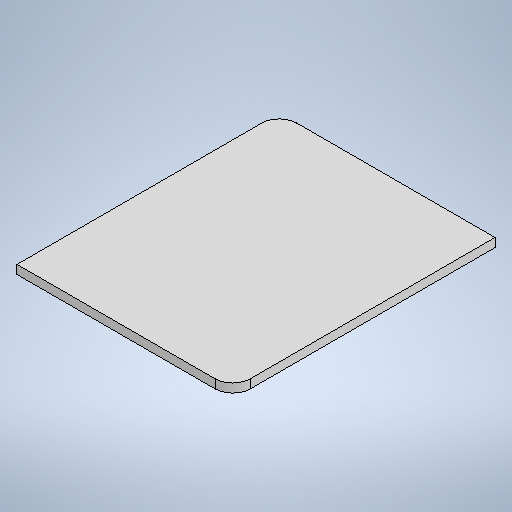
# Autodesk Inventor part: DSB-104 ridge end cap
Saved by Autodesk Inventor 2025.1 (Build 291241020, 241B)
## iProperties
Created: 2025-01-16
Part Number: DSB-104 ridge end cap
Material: Stainless Steel
Document SubType Name: Sheet Metal
Designer: pokla
Density: 8 g/cm^3
Sheet Metal Rule: AISI304 3mm Die 32
Appearance: Default
Mass: 77.6051 g
Surface Area: 103.045 cm^2
Volume: 9.70063 cm^3
Flat Pattern Width: 7.4 cm
Flat Pattern Length: 9 cm
Flat Pattern Area: 66.6 cm^2
Sheet Metal Width: 74.000 mm
Sheet Metal Length: 90.000 mm
Sheet Metal Area: 6660.000 mm^2
Author: pokla
Autodesk Inventor part; units mm, degrees
ref_plane "YZ Plane" through (0, 0, 0) normal (1, 0, 0) x (0, 1, 0)
ref_plane "XZ Plane" through (0, 0, 0) normal (0, 1, 0) x (-1, 0, 0)
ref_plane "XY Plane" through (0, 0, 0) normal (0, 0, 1) x (1, 0, 0)
sketch "Sketch1" plane through (0, 0, 0) normal (0, 0, 1) x (1, 0, 0)
  line L0 (-37, 45) -> (37, 45)
  line L1 (37, 45) -> (37, -45)
  line L2 (37, -45) -> (-37, -45)
  line L3 (-37, -45) -> (-37, 45)
  line L4 (-37, 45) -> (37, -45) construction
  point P0 (0, 0)
  point P1 (0, 0)
  dimension "d0" = 74
  dimension "d1" = 90
  measures "d0" distance of L0.start L0.end
  measures "d1" distance of L2.end L0.start
extrude "Plate1" add sketch "Sketch1" along normal blind 3
fillet "Corner Round2" radius 6 2 edges at (37, -45, 1.5) (-37, 45, 1.5)
equation "\"d2\" = Thickness"
equation "\"BendReliefWidth\" = Thickness"
equation "\"BendReliefDepth\" = 0.5 * Thickness"
equation "\"CornerReliefSize\" = 4 * Thickness"
equation "\"MinimumRemnant\" = 2 * Thickness"
equation "\"TransitionRadius\" = BendRadius"
equation "\"JacobiRadiusSize\" = BendRadius"
equation "\"GapSize\" = Thickness"
equation "\"Thickness\" = 3"
equation "\"BendRadius\" = 5"
body "Solid1"
